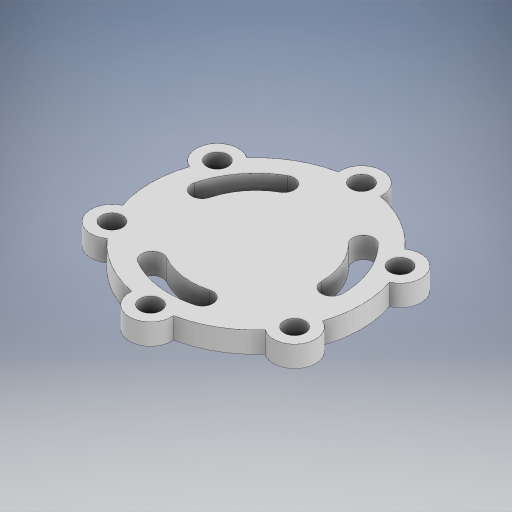
# Autodesk Inventor part: CE-1.3.2
Saved by Autodesk Inventor 2024 (Build 280153000, 153)
## iProperties
Created: 2024-01-25
Part Number: CE-1.3.2
Material: Generic
Document SubType Name: Modeling
Designer: Alex
Density: 1 g/cm^3
Appearance: Default
Author: Alex
Autodesk Inventor part; units mm, degrees
ref_plane "YZ Plane" through (0, 0, 0) normal (1, 0, 0) x (0, 1, 0)
ref_plane "XZ Plane" through (0, 0, 0) normal (0, 1, 0) x (-1, 0, 0)
ref_plane "XY Plane" through (0, 0, 0) normal (0, 0, 1) x (1, 0, 0)
sketch "Sketch1" plane through (0, 0, 0) normal (0, 1, 0) x (-1, 0, 0)
  circle A0 centre (0, 0) radius 36 construction
  circle A1 centre (0, -50) radius 5
  arc A2 (-9.9499, -49) -> (9.9499, -49) centre (0, -50) ccw
  line L0 (0, 0) -> (0, -50) construction
  line L1 (0, 0) -> (25, -43.3013) construction
  line L2 (0, 0) -> (50, 0) construction
  arc A3 (15.5, -26.8468) -> (20.5, -35.507) centre (18, -31.1769) ccw
  line L3 (0, 0) -> (48.2963, -12.941) construction
  line L4 (0, 0) -> (50, 0) construction
  arc A4 (39.603, -10.6116) -> (29.9437, -8.0234) centre (34.7733, -9.3175) ccw
  arc A5 (29.9437, -8.0234) -> (15.5, -26.8468) centre (0, 0) ccw construction
  arc A6 (39.603, -10.6116) -> (20.5, -35.507) centre (0, 0) ccw construction
  arc A7 (20.5, -35.507) -> (39.603, -10.6116) centre (0, 0) ccw
  arc A8 (15.5, -26.8468) -> (29.9437, -8.0234) centre (0, 0) ccw
  circle A9 centre (-43.3013, -25) radius 5
  arc A10 (-47.4102, -15.8832) -> (-37.4603, -33.1168) centre (-43.3013, -25) ccw
  circle A11 centre (-43.3013, 25) radius 5
  arc A12 (-37.4603, 33.1168) -> (-47.4102, 15.8832) centre (-43.3013, 25) ccw
  circle A13 centre (0, 50) radius 5
  arc A14 (9.9499, 49) -> (-9.9499, 49) centre (0, 50) ccw
  circle A15 centre (43.3013, 25) radius 5
  arc A16 (47.4102, 15.8832) -> (37.4603, 33.1168) centre (43.3013, 25) ccw
  circle A17 centre (43.3013, -25) radius 5
  arc A18 (37.4603, -33.1168) -> (47.4102, -15.8832) centre (43.3013, -25) ccw
  arc A19 (15.5, 26.8468) -> (20.5, 35.507) centre (18, 31.1769) ccw
  arc A20 (20.5, 35.507) -> (-10.6116, 39.603) centre (0, 0) ccw
  arc A21 (15.5, 26.8468) -> (-8.0234, 29.9437) centre (0, 0) ccw
  arc A22 (-10.6116, 39.603) -> (-8.0234, 29.9437) centre (-9.3175, 34.7733) ccw
  arc A23 (-31, 0) -> (-41, 0) centre (-36, 0) ccw
  arc A24 (-41, 0) -> (-28.9914, -28.9914) centre (0, 0) ccw
  arc A25 (-31, 0) -> (-21.9203, -21.9203) centre (0, 0) ccw
  arc A26 (-28.9914, -28.9914) -> (-21.9203, -21.9203) centre (-25.4558, -25.4558) ccw
  arc A27 (9.9499, -49) -> (37.4603, -33.1168) centre (0, 0) ccw
  arc A28 (47.4102, -15.8832) -> (47.4102, 15.8832) centre (0, 0) ccw
  arc A29 (37.4603, 33.1168) -> (9.9499, 49) centre (0, 0) ccw
  arc A30 (-9.9499, 49) -> (-37.4603, 33.1168) centre (0, 0) ccw
  arc A31 (-47.4102, 15.8832) -> (-47.4102, -15.8832) centre (0, 0) ccw
  arc A32 (-37.4603, -33.1168) -> (-9.9499, -49) centre (0, 0) ccw
  circle A33 centre (0, 0) radius 50 construction
  dimension "d20" = 100
  dimension "d0" = 72
  dimension "d4" = 10
  dimension "d5" = 10
  dimension "d6" = 60
  dimension "d7" = 10
  dimension "d8" = 15
  dimension "d10" = 10
  dimension "d13" = 360
  dimension "d17" = 360
  dimension "d19" = 50
  constraints: 56 point on circle, 33 centre point, 13 coincident, 10 end point, 2 equal length, 2 horizontal, 2 point on line, 2 tangent, 1 vertical, 1 vertical alignment, 76 other
  measures "d0" diameter of A0
  measures "d4" radius of A2
  measures "d5" diameter of A1
  measures "d6" angle of L1 L2
  measures "d7" diameter of A3
  measures "d8" angle of L3 L4
  measures "d10" diameter of A4
  measures "d19" radius of A32
extrude "Extrusion1" add sketch "Sketch1" along normal blind 10
body "Solid1"
